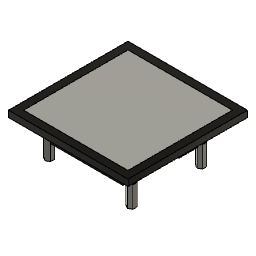
Hyper Pixel 4.0 Square Touch TFT display (Autodesk Fusion 360 design; units mm, degrees)
Autodesk Fusion 360 part; units mm, degrees
sketch "Sketch1" plane through (0, 0, 0) normal (0, 0, 1) x (1, 0, 0)
  line L0 (42, -42) -> (-42, -42)
  line L1 (-42, -42) -> (-42, 42)
  line L2 (-42, 42) -> (42, 42)
  line L3 (42, 42) -> (42, -42)
  line L4 (42, -42) -> (-42, 42) construction
  line L5 (-42, -42) -> (42, 42) construction
  dimension "d1" = 84
  dimension "d2" = 84
  constraint horizontal L0
  constraint perpendicular L0 L1
  constraint parallel L0 L2
  constraint parallel L1 L3
  constraint coincident L4 origin
  constraint coincident L5 origin
  measures "d1" distance of L1.end L2.end
  measures "d2" distance of L0.end L1.end
extrude "Extrude1" add sketch "Sketch1" along normal blind 4.5 makes body 1
sketch "Sketch2" plane through (0, 0, 4.5) normal (0, 0, 1) x (-1, 0, 0)
  line L0 (-42, -42) -> (42, -42)
  line L1 (42, -42) -> (42, 42)
  line L2 (42, 42) -> (-42, 42)
  line L3 (-42, 42) -> (-42, -42)
  line L4 (36.75, -36.75) -> (36.75, 36.75)
  line L5 (36.75, 36.75) -> (-36.75, 36.75)
  line L6 (-36.75, 36.75) -> (-36.75, -36.75)
  line L7 (-36.75, -36.75) -> (36.75, -36.75)
  dimension "d5" = -5.25
split_face "SplitFace1" 1 faces at (-14, -14, 4.5) by curves path "Sketch2" along L4 L5 L6 L7 on bodies 1
sketch "Sketch3" plane through (0, 0, 0) normal (0, 0, -1) x (1, 0, 0)
  line L0 (-42, -42) -> (42, -42)
  line L1 (42, -42) -> (42, 42)
  line L2 (42, 42) -> (-42, 42)
  line L3 (-42, 42) -> (-42, -42)
  line L4 (40.7, 32.75) -> (35.2, 32.75) construction
  line L5 (35.2, 32.75) -> (35.2, 38.25) construction
  line L6 (35.2, 38.25) -> (40.7, 38.25) construction
  line L7 (40.7, 38.25) -> (40.7, 32.75) construction
  line L8 (40.7, 32.75) -> (35.2, 38.25) construction
  line L9 (35.2, 32.75) -> (40.7, 38.25) construction
  circle A0 centre (37.95, 35.5) radius 2.75
  circle A1 centre (-20.05, 35.5) radius 2.75
  line L10 (-17.3, 32.75) -> (-22.8, 32.75) construction
  line L11 (-22.8, 32.75) -> (-22.8, 38.25) construction
  line L12 (-22.8, 38.25) -> (-17.3, 38.25) construction
  line L13 (-17.3, 38.25) -> (-17.3, 32.75) construction
  line L14 (-17.3, 32.75) -> (-22.8, 38.25) construction
  line L15 (-22.8, 32.75) -> (-17.3, 38.25) construction
  circle A2 centre (37.95, -13.5) radius 2.75
  circle A3 centre (-20.05, -13.5) radius 2.75
  circle A4 centre (-20.05, 35.5) radius 1.35
  circle A5 centre (37.95, 35.5) radius 1.35
  circle A6 centre (37.95, -13.5) radius 1.35
  circle A7 centre (-20.05, -13.5) radius 1.35
  point P0 (37.95, 35.5)
  point P1 (-20.05, 35.5)
  dimension "d6" = 3.75
  dimension "d7" = 1.3
  dimension "d8" = 5.5
  dimension "d10" = 58
  dimension "d11" = 49
  dimension "d14" = 2.7
  constraint horizontal L4
  constraint perpendicular L4 L5
  constraint parallel L4 L6
  constraint parallel L5 L7
  constraint coincident L8 P0
  constraint coincident L9 P0
  constraint equal L5 L6
  constraint coincident P0 A0.centre
  constraint tangent L6 A0
  constraint horizontal L10
  constraint perpendicular L10 L11
  constraint parallel L10 L12
  constraint parallel L11 L13
  constraint coincident L14 P1
  constraint coincident L15 P1
  constraint coincident P1 A1.centre
  constraint tangent A1 L12
  constraint tangent A1 L13
  constraint equal A0 A1
  constraint horizontal P0 P1
  constraint equal A0 A2
  constraint equal A0 A3
  constraint vertical P1 A3.centre
  constraint vertical P0 A2.centre
  constraint horizontal A2.centre A3.centre
  constraint concentric A1 A4
  constraint concentric A0 A5
  constraint concentric A2 A6
  constraint concentric A3 A7
  constraint equal A4 A7
  constraint equal A4 A5
  constraint equal A5 A6
  measures "d6" distance of L2 L6
  measures "d7" distance of L1 L7
  measures "d8" distance of L4.end L5.end
  measures "d10" distance of P0 P1
  measures "d11" distance of P1 A3.centre
  measures "d14" diameter of A4
extrude "Extrude2" add sketch "Sketch3" along normal blind 2.18 contours A0 | A1 | A2 | A3 bodies 1
sketch "Sketch4" plane through (0, 0, 0) normal (0, 0, -1) x (1, 0, 0)
  circle A0 centre (37.95, 35.5) radius 2.75
  circle A1 centre (-20.05, 35.5) radius 2.75
  line L0 (-42, -42) -> (42, -42)
  line L1 (42, -42) -> (42, 42)
  line L2 (42, 42) -> (-42, 42)
  line L3 (-42, 42) -> (-42, -42)
  circle A2 centre (-20.05, -13.5) radius 2.75
  circle A3 centre (37.95, -13.5) radius 2.75
  line L4 (37.95, 35.5) -> (-20.05, 35.5) construction
  line L5 (34.6, 38.04) -> (-16.7, 38.04)
  line L6 (-16.7, 38.04) -> (-16.7, 32.96)
  line L7 (-16.7, 32.96) -> (34.6, 32.96)
  line L8 (34.6, 32.96) -> (34.6, 38.04)
  line L9 (34.6, 38.04) -> (-16.7, 32.96) construction
  line L10 (-16.7, 38.04) -> (34.6, 32.96) construction
  point P0 (8.95, 35.5)
  dimension "d17" = 5.08
  dimension "d18" = 51.3
  constraint coincident A0.centre L4.start
  constraint coincident A1.centre L4.end
  constraint horizontal L5
  constraint perpendicular L5 L6
  constraint parallel L5 L7
  constraint parallel L6 L8
  constraint coincident L9 P0
  constraint coincident L10 P0
  constraint midpoint L4 P0
  measures "d17" distance of L5.start L7.end
  measures "d18" distance of L6.end L7.end
extrude "Extrude3" add sketch "Sketch4" along normal blind 5 contours L5 L6 L7 L8 bodies 1
sketch "Sketch5" plane through (0, 0, 0) normal (0, 0, -1) x (1, 0, 0)
  line L0 (34.6, 32.96) -> (-16.7, 32.96)
  line L1 (-16.7, 32.96) -> (-16.7, 38.04)
  line L2 (-16.7, 38.04) -> (34.6, 38.04)
  line L3 (34.6, 38.04) -> (34.6, 32.96)
  circle A0 centre (37.95, 35.5) radius 2.75
  circle A1 centre (-20.05, 35.5) radius 2.75
  line L4 (-42, -42) -> (42, -42)
  line L5 (42, -42) -> (42, 42)
  line L6 (42, 42) -> (-42, 42)
  line L7 (-42, 42) -> (-42, -42)
  circle A2 centre (-20.05, -13.5) radius 2.75
  circle A3 centre (37.95, -13.5) radius 2.75
  line L8 (30.79, -9.76) -> (38.94, -9.76)
  line L9 (38.94, -9.76) -> (38.94, 3.09)
  line L10 (38.94, 3.09) -> (30.79, 3.09)
  line L11 (30.79, 3.09) -> (30.79, -9.76)
  line L12 (30.79, -9.76) -> (38.94, 3.09) construction
  line L13 (38.94, -9.76) -> (30.79, 3.09) construction
  point P0 (34.865, -3.335)
  dimension "d21" = 12.85
  dimension "d22" = 8.15
  dimension "d23" = 45.09
  dimension "d24" = 3.06
  constraint horizontal L8
  constraint perpendicular L8 L9
  constraint parallel L8 L10
  constraint parallel L9 L11
  constraint coincident L12 P0
  constraint coincident L13 P0
  measures "d21" distance of L8.start L10.end
  measures "d22" distance of L9.end L10.end
  measures "d23" distance of L4 L10
  measures "d24" distance of L5 L9
extrude "Extrude4" add sketch "Sketch5" along normal blind 3.71 contours L8 L9 L10 L11 bodies 1
sketch "Sketch1 (2)" plane through (0, 0, -2.18) normal (0, 0, -1) x (1, 0, 0) in component "Standoffs"
  circle A0 centre (-20.05, -13.5) radius 1.35
  circle A1 centre (-20.05, -13.5) radius 2.75
  line L0 (-17.55, -14.9434) -> (-17.55, -12.0566)
  line L1 (-17.55, -12.0566) -> (-20.05, -10.6132)
  line L2 (-20.05, -10.6132) -> (-22.55, -12.0566)
  line L3 (-22.55, -12.0566) -> (-22.55, -14.9434)
  line L4 (-22.55, -14.9434) -> (-20.05, -16.3868)
  line L5 (-20.05, -16.3868) -> (-17.55, -14.9434)
  line L6 (-20.05, -13.5) -> (-20.05, -25) construction
  circle A2 centre (-20.05, -13.5) radius 1.35
  circle A3 centre (-20.05, 35.5) radius 1.35
  circle A4 centre (37.95, 35.5) radius 1.35
  circle A5 centre (37.95, -13.5) radius 1.35
  line L7 (-20.05, 35.5) -> (37.95, 35.5) construction
  line L8 (37.95, 35.5) -> (37.95, -13.5) construction
  line L9 (8.95, 35.5) -> (8.95, -25) construction
  line L10 (37.95, 11) -> (-20, 11) construction
  line L11 (-17.55, 34.0566) -> (-20.05, 32.6132)
  line L12 (-20.05, 32.6132) -> (-22.55, 34.0566)
  line L13 (-17.55, 36.9434) -> (-17.55, 34.0566)
  line L14 (-20.05, 38.3868) -> (-17.55, 36.9434)
  line L15 (-22.55, 36.9434) -> (-20.05, 38.3868)
  line L16 (-22.55, 34.0566) -> (-22.55, 36.9434)
  circle A6 centre (-20.05, 35.5) radius 1.35
  line L17 (35.45, 34.0566) -> (37.95, 32.6132)
  line L18 (35.45, 36.9434) -> (35.45, 34.0566)
  line L19 (37.95, 38.3868) -> (35.45, 36.9434)
  line L20 (40.45, 36.9434) -> (37.95, 38.3868)
  line L21 (40.45, 34.0566) -> (40.45, 36.9434)
  line L22 (37.95, 32.6132) -> (40.45, 34.0566)
  line L23 (35.45, -12.0566) -> (37.95, -10.6132)
  line L24 (37.95, -10.6132) -> (40.45, -12.0566)
  line L25 (40.45, -12.0566) -> (40.45, -14.9434)
  line L26 (35.45, -14.9434) -> (35.45, -12.0566)
  line L27 (37.95, -16.3868) -> (35.45, -14.9434)
  line L28 (40.45, -14.9434) -> (37.95, -16.3868)
  circle A7 centre (37.95, -13.5) radius 1.35
  circle A8 centre (37.95, 35.5) radius 1.35
  point P0 (-20.05, -13.5)
  dimension "d27" = 2.5
  constraint coincident P0 A0.centre
  constraint vertical L6
  constraint coincident L4.end L6
  constraint coincident A3.centre L7.start
  constraint coincident A4.centre L7.end
  constraint coincident A5.centre L8.end
  constraint midpoint L7 L9.start
  constraint perpendicular L7 L9
  constraint midpoint L8 L10.start
  constraint perpendicular L8 L10
  constraint symmetric L0.start L10 L13.start
  constraint symmetric L0.end L10 L11.start
  constraint symmetric L1.end L10 L11.end
  constraint symmetric L2.end L10 L12.end
  constraint symmetric L3.end L10 L15.start
  constraint symmetric L4.end L10 L14.start
  constraint symmetric A2 L10 A6
  constraint symmetric L0.start L9 L26.start
  constraint symmetric L0.end L9 L23.start
  constraint symmetric L1.end L9 L23.end
  constraint symmetric L2.end L9 L24.end
  constraint symmetric L3.end L9 L25.end
  constraint symmetric L4.end L9 L27.start
  constraint symmetric A2 L9 A7
  constraint symmetric L9 L11.start L17.start
  constraint symmetric L9 L11.end L17.end
  constraint symmetric L9 L12.end L21.start
  constraint symmetric L9 L13.start L18.start
  constraint symmetric L9 L14.start L19.start
  constraint symmetric L9 L15.start L20.start
  constraint symmetric L9 A6 A8
  measures "d27" distance of P0 L5
extrude "Extrude1'" add sketch "Sketch1 (2)" along normal blind 15 separate body contours A1 L0 L1 L2 L3 L4 L5 | L11 L12 L13 L14 L15 L16 | L17 L18 L19 L20 L21 L22 | L23 L24 L25 L26 L27 L28 makes body 2 at (-21.3933, -35.3656, -12.18) makes body 3 at (38.5659, 12.2987, -12.18) makes body 4 at (37.3341, -36.7013, -12.18) makes body 5 at (-18.7067, 13.6344, -12.18) in component "Standoffs"
component "Standoffs" placed x (1, 0, 0) y (0, 1, 0) z (0, 0, 1) at (0, 0, 0)
equation "d27 = ( 5 / 2 ) * 1 mm"
